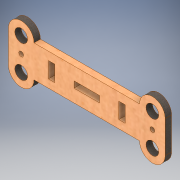
# Autodesk Inventor part: PistonPart1
Saved by Autodesk Inventor 2019 (Build 230136000, 136)
## iProperties
Created: 2021-01-03
Part Number: PistonPart1
Material: Дерево (вишня)
Document SubType Name: Modeling
Designer: Professional
Density: 0.63 g/cm^3
Appearance: Вишневое дерево — натуральный — со слабым глянцем
Author: Professional
Autodesk Inventor part; units mm, degrees
ref_plane "YZ Plane" through (0, 0, 0) normal (1, 0, 0) x (0, 1, 0)
ref_plane "XZ Plane" through (0, 0, 0) normal (0, 1, 0) x (-1, 0, 0)
ref_plane "XY Plane" through (0, 0, 0) normal (0, 0, 1) x (1, 0, 0)
sketch "Эскиз1" plane through (0, 0, 0) normal (0, 0, 1) x (1, 0, 0)
  circle A0 centre (-41, -10) radius 4
  circle A1 centre (-41, 10) radius 4
  circle A2 centre (41, 10) radius 4
  circle A3 centre (41, -10) radius 4
  line L0 (-41, 10) -> (41, 10) construction
  line L1 (41, 10) -> (41, -10) construction
  line L2 (41, -10) -> (-41, -10) construction
  line L3 (-41, -10) -> (-41, 10) construction
  arc A4 (-33, 10) -> (-49, 10) centre (-41, 10) ccw
  arc A5 (-49, -10) -> (-33, -10) centre (-41, -10) ccw
  arc A6 (33, -10) -> (49, -10) centre (41, -10) ccw
  arc A7 (49, 10) -> (33, 10) centre (41, 10) ccw
  line L4 (-49, 10) -> (-49, -10)
  line L5 (49, 10) -> (49, -10)
  line L6 (33, 10) -> (-33, 10)
  line L7 (33, -10) -> (-33, -10)
  line L8 (8, -2) -> (-8, -2)
  line L9 (-8, -2) -> (-8, 2)
  line L10 (-8, 2) -> (8, 2)
  line L11 (8, 2) -> (8, -2)
  line L12 (24, 5) -> (20, 5)
  line L13 (20, 5) -> (20, -5)
  line L14 (20, -5) -> (24, -5)
  line L15 (24, -5) -> (24, 5)
  line L16 (0, 10) -> (0, -10)
  line L17 (-24, 5) -> (-20, 5)
  line L18 (-20, 5) -> (-20, -5)
  line L19 (-20, -5) -> (-24, -5)
  line L20 (-24, -5) -> (-24, 5)
  point P0 (0, 0)
  point P1 (41, 0)
  point P2 (0, 2)
  point P3 (8, 0)
  point P4 (20, 0)
  point P5 (-20, 0)
  dimension "d0" = 8
  dimension "d1" = 20
  dimension "d2" = 82
  dimension "d3" = 8
  dimension "d6" = 10
  dimension "d7" = 10
  dimension "d8" = 4
  dimension "d9" = 16
  dimension "d10" = 10
  dimension "d11" = 40
  constraints: 42 end point, 9 point on circle, 8 centre point, 6 equal radius, 6 midpoint, 6 parallel, 5 horizontal, 5 horizontal alignment, 5 symmetric about line, 4 coincident, 4 perpendicular, 4 vertical alignment, 2 tangent, 2 vertical, 1 point on line
  measures "d0" diameter of A1
  measures "d1" distance of L0.start A0.centre
  measures "d2" distance of A2.centre L0.start
  measures "d3" radius of A7
  measures "d6" distance from line of point (0, 0) L6
  measures "d7" distance from line of L7 point (0, 0)
  measures "d8" distance between parallel lines of L10 L8
  measures "d9" distance between parallel lines of L9 L11
  measures "d10" distance of L12.end L13.end
  measures "d11" distance between parallel lines of L18 L13
extrude "Выдавливание1" add sketch "Эскиз1" along normal blind 4 contours L6 L16 L10 L9 L8 L7 A5 L4 A4 | L6 A7 L5 A6 L7 L16 L8 L11 L10
sketch "Эскиз2" plane through (0, 0, 4) normal (0, 0, 1) x (1, 0, 0)
  line L0 (-8, -2) -> (-8, 2) projected
  line L1 (-8, 2) -> (8, 2) projected
  line L2 (8, 2) -> (8, -2) projected
  line L3 (8, -2) -> (-8, -2) projected
  circle A0 centre (41, -10) radius 4 projected
  circle A1 centre (41, 10) radius 4 projected
  circle A2 centre (-41, 10) radius 4 projected
  circle A3 centre (-41, -10) radius 4 projected
  line L4 (-20, 5) -> (-20, -5) projected
  line L5 (-20, -5) -> (-24, -5) projected
  line L6 (-24, -5) -> (-24, 5) projected
  line L7 (-24, 5) -> (-20, 5) projected
  line L8 (24, 5) -> (24, -5) projected
  line L9 (24, -5) -> (20, -5) projected
  line L10 (20, -5) -> (20, 5) projected
  line L11 (20, 5) -> (24, 5) projected
  arc A4 (-33, 10) -> (-49, 10) centre (-41, 10) ccw projected
  line L12 (-49, 10) -> (-49, -10) projected
  arc A5 (-49, -10) -> (-33, -10) centre (-41, -10) ccw projected
  line L13 (-33, -10) -> (33, -10) projected
  arc A6 (33, -10) -> (49, -10) centre (41, -10) ccw projected
  line L14 (49, -10) -> (49, 10) projected
  arc A7 (49, 10) -> (33, 10) centre (41, 10) ccw projected
  line L15 (33, 10) -> (-33, 10) projected
  point P0 (0, 0)
  point P1 (41, 0)
  point P2 (-41, 0)
  constraints: 2 horizontal alignment, 2 vertical alignment
hole "Отверстие1" at (41, 0, 4) at (-41, 0, 4) direction (0, 0, -1) diameter 3 end through all
